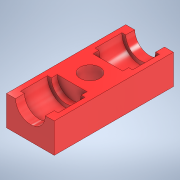
# Autodesk Inventor part: Mancal sup dos motores
Saved by Autodesk Inventor 2021 (Build 250183000, 183)
## iProperties
Created: 2021-11-17
Part Number: Mancal sup dos motores
Material: Generic
Document SubType Name: Modeling
Designer: Matheus
Density: 1 g/cm^3
Appearance: Light Red
Author: Matheus
Autodesk Inventor part; units mm, degrees
ref_plane "YZ Plane" through (0, 0, 0) normal (1, 0, 0) x (0, 1, 0)
ref_plane "XZ Plane" through (0, 0, 0) normal (0, 1, 0) x (-1, 0, 0)
ref_plane "XY Plane" through (0, 0, 0) normal (0, 0, 1) x (1, 0, 0)
sketch "Sketch1" plane through (0, 0, 0) normal (0, 0, 1) x (1, 0, 0)
  line L0 (0, -1) -> (0, 6) construction
  line L1 (4, 0) -> (-4, 0)
  line L2 (-4, 0) -> (-4, 5)
  line L3 (-4, 5) -> (4, 5)
  line L4 (4, 5) -> (4, 0)
  line L5 (-5.6, 0) -> (5.6, 0) construction
  point P0 (0, 0)
  dimension "d0" = 5
  dimension "d1" = 8
  constraints: 8 end point, 2 parallel, 1 collinear, 1 horizontal, 1 perpendicular, 1 other
  measures "d0" distance of L1.end L2.end
  measures "d1" distance of L2.end L3.end
extrude "Extrusion1" add sketch "Sketch1" along normal mid plane 20
sketch "Sketch2" plane through (0, 0, 10) normal (0, 0, 1) x (1, 0, 0)
  line L0 (0, -1) -> (0, 6) construction
  line L1 (-5.6, 0) -> (5.6, 0) construction
  line L2 (4, 5) -> (-4, 5) construction
  arc A0 (-2.5, 5) -> (2.5, 5) centre (0, 5) ccw
  line L3 (-2.5, 5) -> (2.5, 5)
  point P0 (0, 0)
  dimension "d4" = 5
  constraints: 2 end point, 2 point on circle, 2 point on line, 1 centre point, 1 midpoint
  measures "d4" diameter of A0
extrude "Extrusion2" cut sketch "Sketch2" against normal blind 7
ref_plane "Work Plane1" through (0, 0, 8.5) normal (0, 0, 1) x (1, 0, 0)
sketch "Sketch3" plane through (0, 0, 8.5) normal (0, 0, 1) x (1, 0, 0)
  line L0 (0, -1.63) -> (0, 9.78) construction
  circle A0 centre (0, 5) radius 3.15
  line L1 (4, 5) -> (2.5, 5) construction
  point P0 (0, 0)
  dimension "d8" = 6.3
  constraints: 2 point on line, 1 centre point
  measures "d8" diameter of A0
extrude "Extrusion3" cut sketch "Sketch3" against normal blind 4.5
mirror "Mirror2" about plane through (0, 0, 0) normal (0, 0, 1) of "Extrusion3", "Extrusion2"
sketch "Sketch4" plane through (-4, 5, 10) normal (0, 1, 0) x (1, 0, 0)
  line L0 (9.6, 10) -> (-1.6, 10) construction
  line L1 (4, 24) -> (4, -4) construction
  circle A0 centre (4, 10) radius 1.65
  dimension "d12" = 3.3
  constraints: 1 centre point, 1 coincident
  measures "d12" diameter of A0
extrude "Extrusion4" cut sketch "Sketch4" against normal up to next
sketch "Sketch5" plane through (0, 0, 10) normal (0, 0, 1) x (1, 0, 0)
  line L0 (-4, 0) -> (4, 0) construction
  line L1 (-5.274, 10.3) -> (-17.574, 10.3)
  line L2 (-17.574, 10.3) -> (-17.574, 0)
  line L3 (-17.574, 0) -> (-25, 0)
  line L4 (-25, 0) -> (-25, 2)
  line L5 (-25, 2) -> (-19.574, 2)
  line L6 (-19.574, 2) -> (-19.574, 12.3)
  line L7 (-19.574, 12.3) -> (-4.274, 12.3)
  line L8 (-4, 0) -> (-5.274, 0)
  line L9 (-4, 5) -> (-4, 0) projected
  arc A0 (-2.5, 5) -> (2.5, 5) centre (0, 5) ccw construction
  line L10 (-5.274, 0) -> (-5.274, 10.3)
  line L11 (-11.424, 10.3) -> (-11.424, 0.2772) construction
  line L12 (-4.274, 12.3) -> (-4.274, 5)
  line L13 (-4, 0) -> (-4, 5) construction
  line L14 (-4, 5) -> (-4.274, 5)
  line L15 (-2.5, 5) -> (-4, 5) construction
  point P0 (0, 0)
  point P1 (-5, 0)
  dimension "d16" = 10.3
  dimension "d17" = 12.3
  dimension "d18" = 11.424
  dimension "d19" = 2
  dimension "d20" = 2
  dimension "d21" = 2
  dimension "d22" = 25
  dimension "d23" = 1
  constraints: 26 end point, 6 perpendicular, 4 vertical, 3 collinear, 1 horizontal, 1 midpoint, 1 point on line
  measures "d16" distance of L1.end L2.end
  measures "d17" distance of L1.start L1.end
  measures "d18" distance from line of A0.centre L11
  measures "d19" distance between parallel lines of L2 L6
  measures "d20" distance between parallel lines of L1 L7
  measures "d21" distance between parallel lines of L3 L5
  measures "d22" distance from line of point (0, 0) L4
  measures "d23" distance between parallel lines of L10 L12
body "Solid1"
